Autodesk Inventor part; units mm, degrees
note: some values were not read from the file. Chosen so that the rebuilt part matches the saved one: direction of "Emboss2".
(part 2 of 2)
  line L273 (-8.8546, 3.3987) -> (-8.8546, 3.6622)
  line L274 (-8.8546, 3.6622) -> (-6.5657, 3.6622)
  line L275 (-6.5657, 3.6622) -> (-6.5657, 4.1129)
  line L276 (-6.5657, 4.1129) -> (-6.3064, 4.1129)
  line L277 (-7.1791, 6.2145) -> (-7.1791, 5.9119)
  line L278 (-7.1791, 5.9119) -> (-6.3064, 5.9119)
  line L279 (-6.3064, 5.9119) -> (-6.3064, 5.5846)
  line L280 (-6.3064, 5.5846) -> (-7.1791, 5.5846)
  line L281 (-7.1791, 5.5846) -> (-7.1791, 4.4628)
  line L282 (-7.1791, 4.4628) -> (-7.5373, 4.4628)
  line L283 (-7.5373, 4.4628) -> (-8.8464, 5.5991)
  line L284 (-8.8464, 5.5991) -> (-8.8464, 5.9119)
  line L285 (-8.8464, 5.9119) -> (-7.4529, 5.9119)
  line L286 (-7.4529, 5.9119) -> (-7.4529, 6.2145)
  line L287 (-7.4529, 6.2145) -> (-7.1791, 6.2145)
  line L288 (-7.4529, 5.5846) -> (-8.445, 5.5846)
  line L289 (-8.445, 5.5846) -> (-7.4529, 4.7304)
  line L290 (-7.4529, 4.7304) -> (-7.4529, 5.5846)
  spline S251 degree 2 poles (-7.5764, 8.067) (-6.893, 8.067) (-6.2529, 7.6698) (-6.2529, 7.256) knots 0 0 0 1 2 2 2
  spline S252 degree 2 poles (-6.2529, 7.256) (-6.2529, 6.8361) (-6.9054, 6.443) (-7.5743, 6.443) knots 0 0 0 1 2 2 2
  spline S253 degree 2 poles (-7.5743, 6.443) (-8.2618, 6.443) (-8.8978, 6.8402) (-8.8978, 7.256) knots 0 0 0 1 2 2 2
  spline S254 degree 2 poles (-8.8978, 7.256) (-8.8978, 7.6739) (-8.2392, 8.067) (-7.5764, 8.067) knots 0 0 0 1 2 2 2
  spline S255 degree 2 poles (-6.8024, 7.6306) (-6.928, 7.68) (-7.315, 7.7212) (-7.5764, 7.7212) knots 0 0 0 1 2 2 2
  spline S256 degree 2 poles (-7.5764, 7.7212) (-7.8378, 7.7212) (-8.2227, 7.68) (-8.3524, 7.6286) knots 0 0 0 1 2 2 2
  spline S257 degree 2 poles (-8.3524, 7.6286) (-8.4821, 7.5771) (-8.6158, 7.3981) (-8.6158, 7.256) knots 0 0 0 1 2 2 2
  spline S258 degree 2 poles (-8.6158, 7.256) (-8.6158, 7.114) (-8.4821, 6.9308) (-8.3483, 6.8773) knots 0 0 0 1 2 2 2
  spline S259 degree 2 poles (-8.3483, 6.8773) (-8.2186, 6.8258) (-7.8234, 6.7888) (-7.5743, 6.7888) knots 0 0 0 1 2 2 2
  spline S260 degree 2 poles (-7.5743, 6.7888) (-7.3067, 6.7888) (-6.9486, 6.8217) (-6.8086, 6.8752) knots 0 0 0 1 2 2 2
  spline S261 degree 2 poles (-6.8086, 6.8752) (-6.6769, 6.9246) (-6.5349, 7.1078) (-6.5349, 7.256) knots 0 0 0 1 2 2 2
  spline S262 degree 2 poles (-6.5349, 7.256) (-6.5349, 7.396) (-6.6687, 7.5792) (-6.8024, 7.6306) knots 0 0 0 1 2 2 2
  point P0 (0, 0)
  constraints: 22 other
emboss "Emboss2" sketch "Sketch2" operation cut depth 0.762 direction (0, -1, 0)
body "Solid2"
